Autodesk Fusion 360 part; units mm, degrees
note: some values were not read from the file. Chosen so that the rebuilt part matches the saved one: which face or edge a step refers to.
(part 3 of 3)
sketch "Sketch7" plane through (0, -7, 0) normal (0, -1, 0) x (1, 0, 0)
  circle A0 centre (0, 0) radius 34.5
  circle A1 centre (0, 0) radius 49
  line L0 (0, 34.5) -> (0, 36.5)
  line L1 (0, 36.5) -> (0, 37.03)
  line L2 (0, 37.03) -> (3.25, 37.03)
  line L3 (3.25, 37.03) -> (3.25, 34.3466)
  line L4 (-6.3382, 35.9455) -> (-6.4302, 36.4674)
  line L5 (-6.4302, 36.4674) -> (-3.2296, 37.0318)
  line L6 (-3.2296, 37.0318) -> (-2.7636, 34.3891)
  line L7 (-5.9909, 33.9759) -> (-6.3382, 35.9455)
  line L8 (-12.4837, 34.2988) -> (-12.665, 34.7968)
  line L9 (-12.665, 34.7968) -> (-9.611, 35.9084)
  line L10 (-9.611, 35.9084) -> (-8.6932, 33.3868)
  line L11 (-11.7997, 32.4194) -> (-12.4837, 34.2988)
  line L12 (-18.25, 31.6099) -> (-18.515, 32.0689)
  line L13 (-18.515, 32.0689) -> (-15.7004, 33.6939)
  line L14 (-15.7004, 33.6939) -> (-14.3587, 31.37)
  line L15 (-17.25, 29.8779) -> (-18.25, 31.6099)
  line L16 (-23.4617, 27.9606) -> (-23.8024, 28.3666)
  line L17 (-23.8024, 28.3666) -> (-21.3128, 30.4557)
  line L18 (-21.3128, 30.4557) -> (-19.5879, 28.4001)
  line L19 (-22.1762, 26.4285) -> (-23.4617, 27.9606)
  line L20 (-27.9606, 23.4617) -> (-28.3666, 23.8024)
  line L21 (-28.3666, 23.8024) -> (-26.2776, 26.2921)
  line L22 (-26.2776, 26.2921) -> (-24.2219, 24.5672)
  line L23 (-26.4285, 22.1762) -> (-27.9606, 23.4617)
  line L24 (-31.6099, 18.25) -> (-32.0689, 18.515)
  line L25 (-32.0689, 18.515) -> (-30.4439, 21.3296)
  line L26 (-30.4439, 21.3296) -> (-28.12, 19.9879)
  line L27 (-29.8779, 17.25) -> (-31.6099, 18.25)
  line L28 (-34.2988, 12.4837) -> (-34.7968, 12.665)
  line L29 (-34.7968, 12.665) -> (-33.6853, 15.719)
  line L30 (-33.6853, 15.719) -> (-31.1637, 14.8012)
  line L31 (-32.4194, 11.7997) -> (-34.2988, 12.4837)
  line L32 (-35.9455, 6.3382) -> (-36.4674, 6.4302)
  line L33 (-36.4674, 6.4302) -> (-35.9031, 9.6308)
  line L34 (-35.9031, 9.6308) -> (-33.2604, 9.1648)
  line L35 (-33.9759, 5.9909) -> (-35.9455, 6.3382)
  line L36 (-36.5, 0) -> (-37.03, 0)
  line L37 (-37.03, 0) -> (-37.03, 3.25)
  line L38 (-37.03, 3.25) -> (-34.3466, 3.25)
  line L39 (-34.5, 0) -> (-36.5, 0)
  line L40 (-35.9455, -6.3382) -> (-36.4674, -6.4302)
  line L41 (-36.4674, -6.4302) -> (-37.0318, -3.2296)
  line L42 (-37.0318, -3.2296) -> (-34.3891, -2.7636)
  line L43 (-33.9759, -5.9909) -> (-35.9455, -6.3382)
  line L44 (-34.2988, -12.4837) -> (-34.7968, -12.665)
  line L45 (-34.7968, -12.665) -> (-35.9084, -9.611)
  line L46 (-35.9084, -9.611) -> (-33.3868, -8.6932)
  line L47 (-32.4194, -11.7997) -> (-34.2988, -12.4837)
  line L48 (-31.6099, -18.25) -> (-32.0689, -18.515)
  line L49 (-32.0689, -18.515) -> (-33.6939, -15.7004)
  line L50 (-33.6939, -15.7004) -> (-31.37, -14.3587)
  line L51 (-29.8779, -17.25) -> (-31.6099, -18.25)
  line L52 (-27.9606, -23.4617) -> (-28.3666, -23.8024)
  line L53 (-28.3666, -23.8024) -> (-30.4557, -21.3128)
  line L54 (-30.4557, -21.3128) -> (-28.4001, -19.5879)
  line L55 (-26.4285, -22.1762) -> (-27.9606, -23.4617)
  line L56 (-23.4617, -27.9606) -> (-23.8024, -28.3666)
  line L57 (-23.8024, -28.3666) -> (-26.2921, -26.2776)
  line L58 (-26.2921, -26.2776) -> (-24.5672, -24.2219)
  line L59 (-22.1762, -26.4285) -> (-23.4617, -27.9606)
  line L60 (-18.25, -31.6099) -> (-18.515, -32.0689)
  line L61 (-18.515, -32.0689) -> (-21.3296, -30.4439)
  line L62 (-21.3296, -30.4439) -> (-19.9879, -28.12)
  line L63 (-17.25, -29.8779) -> (-18.25, -31.6099)
  line L64 (-12.4837, -34.2988) -> (-12.665, -34.7968)
  line L65 (-12.665, -34.7968) -> (-15.719, -33.6853)
  line L66 (-15.719, -33.6853) -> (-14.8012, -31.1637)
  line L67 (-11.7997, -32.4194) -> (-12.4837, -34.2988)
  line L68 (-6.3382, -35.9455) -> (-6.4302, -36.4674)
  line L69 (-6.4302, -36.4674) -> (-9.6308, -35.9031)
  line L70 (-9.6308, -35.9031) -> (-9.1648, -33.2604)
  line L71 (-5.9909, -33.9759) -> (-6.3382, -35.9455)
  line L72 (0, -36.5) -> (0, -37.03)
  line L73 (0, -37.03) -> (-3.25, -37.03)
  line L74 (-3.25, -37.03) -> (-3.25, -34.3466)
  line L75 (0, -34.5) -> (0, -36.5)
  line L76 (6.3382, -35.9455) -> (6.4302, -36.4674)
  line L77 (6.4302, -36.4674) -> (3.2296, -37.0318)
  line L78 (3.2296, -37.0318) -> (2.7636, -34.3891)
  line L79 (5.9909, -33.9759) -> (6.3382, -35.9455)
  line L80 (12.4837, -34.2988) -> (12.665, -34.7968)
  line L81 (12.665, -34.7968) -> (9.611, -35.9084)
  line L82 (9.611, -35.9084) -> (8.6932, -33.3868)
  line L83 (11.7997, -32.4194) -> (12.4837, -34.2988)
  line L84 (18.25, -31.6099) -> (18.515, -32.0689)
  line L85 (18.515, -32.0689) -> (15.7004, -33.6939)
  line L86 (15.7004, -33.6939) -> (14.3587, -31.37)
  line L87 (17.25, -29.8779) -> (18.25, -31.6099)
  line L88 (23.4617, -27.9606) -> (23.8024, -28.3666)
  line L89 (23.8024, -28.3666) -> (21.3128, -30.4557)
  line L90 (21.3128, -30.4557) -> (19.5879, -28.4001)
  line L91 (22.1762, -26.4285) -> (23.4617, -27.9606)
  line L92 (27.9606, -23.4617) -> (28.3666, -23.8024)
  line L93 (28.3666, -23.8024) -> (26.2776, -26.2921)
  line L94 (26.2776, -26.2921) -> (24.2219, -24.5672)
  line L95 (26.4285, -22.1762) -> (27.9606, -23.4617)
  line L96 (31.6099, -18.25) -> (32.0689, -18.515)
  line L97 (32.0689, -18.515) -> (30.4439, -21.3296)
  line L98 (30.4439, -21.3296) -> (28.12, -19.9879)
  line L99 (29.8779, -17.25) -> (31.6099, -18.25)
  line L100 (34.2988, -12.4837) -> (34.7968, -12.665)
  line L101 (34.7968, -12.665) -> (33.6853, -15.719)
  line L102 (33.6853, -15.719) -> (31.1637, -14.8012)
  line L103 (32.4194, -11.7997) -> (34.2988, -12.4837)
  line L104 (35.9455, -6.3382) -> (36.4674, -6.4302)
  line L105 (36.4674, -6.4302) -> (35.9031, -9.6308)
  line L106 (35.9031, -9.6308) -> (33.2604, -9.1648)
  line L107 (33.9759, -5.9909) -> (35.9455, -6.3382)
  line L108 (36.5, 0) -> (37.03, 0)
  line L109 (37.03, 0) -> (37.03, -3.25)
  line L110 (37.03, -3.25) -> (34.3466, -3.25)
  line L111 (34.5, 0) -> (36.5, 0)
  line L112 (35.9455, 6.3382) -> (36.4674, 6.4302)
  line L113 (36.4674, 6.4302) -> (37.0318, 3.2296)
  line L114 (37.0318, 3.2296) -> (34.3891, 2.7636)
  line L115 (33.9759, 5.9909) -> (35.9455, 6.3382)
  line L116 (34.2988, 12.4837) -> (34.7968, 12.665)
  line L117 (34.7968, 12.665) -> (35.9084, 9.611)
  line L118 (35.9084, 9.611) -> (33.3868, 8.6932)
  line L119 (32.4194, 11.7997) -> (34.2988, 12.4837)
  line L120 (31.6099, 18.25) -> (32.0689, 18.515)
  line L121 (32.0689, 18.515) -> (33.6939, 15.7004)
  line L122 (33.6939, 15.7004) -> (31.37, 14.3587)
  line L123 (29.8779, 17.25) -> (31.6099, 18.25)
  line L124 (27.9606, 23.4617) -> (28.3666, 23.8024)
  line L125 (28.3666, 23.8024) -> (30.4557, 21.3128)
  line L126 (30.4557, 21.3128) -> (28.4001, 19.5879)
  line L127 (26.4285, 22.1762) -> (27.9606, 23.4617)
  line L128 (23.4617, 27.9606) -> (23.8024, 28.3666)
  line L129 (23.8024, 28.3666) -> (26.2921, 26.2776)
  line L130 (26.2921, 26.2776) -> (24.5672, 24.2219)
  line L131 (22.1762, 26.4285) -> (23.4617, 27.9606)
  line L132 (18.25, 31.6099) -> (18.515, 32.0689)
  line L133 (18.515, 32.0689) -> (21.3296, 30.4439)
  line L134 (21.3296, 30.4439) -> (19.9879, 28.12)
  line L135 (17.25, 29.8779) -> (18.25, 31.6099)
  line L136 (12.4837, 34.2988) -> (12.665, 34.7968)
  line L137 (12.665, 34.7968) -> (15.719, 33.6853)
  line L138 (15.719, 33.6853) -> (14.8012, 31.1637)
  line L139 (11.7997, 32.4194) -> (12.4837, 34.2988)
  line L140 (6.3382, 35.9455) -> (6.4302, 36.4674)
  line L141 (6.4302, 36.4674) -> (9.6308, 35.9031)
  line L142 (9.6308, 35.9031) -> (9.1648, 33.2604)
  line L143 (5.9909, 33.9759) -> (6.3382, 35.9455)
  dimension "d60" = 3.25
  dimension "d62" = 360
  constraint coincident A0 L0.start
  constraint vertical L0
  constraint parallel L0 L1
  constraint perpendicular L1 L2
  constraint coincident A0 L3.end
  constraint perpendicular L2 L3
  measures "d60" distance of L1.end L2.end
sketch "Sketch8" plane through (-23.8024, 0, -28.3666) normal (0.642788, 0, 0.766044) x (0.766044, 0, -0.642788)
  line L0 (-3.25, -7) -> (0, -7)
  line L1 (0, -7) -> (0, 0)
  line L2 (0, 0) -> (-3.25, 0)
  line L3 (-3.25, 0) -> (-3.25, -7)
  line L4 (-3.25, -7) -> (0, -7)
  line L5 (0, -7) -> (0, -2.2084)
  line L6 (-1, -1.2084) -> (-2.25, -1.2084)
  line L7 (-3.25, -2.2084) -> (-3.25, -7)
  arc A0 (-2.25, -1.2084) -> (-3.25, -2.2084) centre (-2.25, -2.2084) ccw
  arc A1 (0, -2.2084) -> (-1, -1.2084) centre (-1, -2.2084) ccw
  dimension "d65" = 1
  dimension "d66" = 5.7916
  constraint horizontal L4
  constraint vertical L5
  constraint horizontal L6
  constraint vertical L7
  constraint tangent L6 A0
  constraint tangent L7 A0
  constraint tangent L6 A1
  constraint tangent L5 A1
  constraint equal A0 A1
  measures "d65" radius of A0
  measures "d66" distance of L4 L6
extrude "Extrude9" cut sketch "Sketch8" along normal blind 6 and the other way blind 22 contours L0 L1 L3 L4 L5 L6 L7 A0 A1
pattern_circular "C-Pattern1" count 36 over 360 about axis through (0, 1.75, 0) along (0, 1, 0) of "Extrude9"
sketch "Sketch9" plane through (0, -7, 0) normal (0, -1, 0) x (1, 0, 0)
  line L0 (0, 34.5) -> (0, 49)
  arc A0 (0, 49) -> (-5.2894, 48.7137) centre (0, 0) ccw
  line L1 (-5.2894, 48.7137) -> (-2.7636, 34.3891)
  arc A1 (0, 34.5) -> (-2.7636, 34.3891) centre (0, 0) ccw
  circle A2 centre (0, 0) radius 49.0012
  circle A3 centre (0, 0) radius 34.5
  dimension "d73" = 69
  constraint concentric A0 A2
  constraint concentric A2 A3
  measures "d73" diameter of A3
extrude "Extrude10" add sketch "Sketch9" along normal blind 1 contours L0 A0 L1 A1 A2 A3 | L0 L1 A2 A3
sketch "Sketch10" plane through (0, -8, 0) normal (0, -1, 0) x (1, 0, 0)
  circle A0 centre (0, 0) radius 34.5
  circle A1 centre (0, 0) radius 49.0012
  circle A2 centre (0, 0) radius 49.0012
  constraint concentric A0 A2
ref_plane "WorkPlane1" through (0, -15, 0) normal (0, -1, 0) x (1, 0, 0)
sketch "Sketch11" plane through (0, -15, 0) normal (0, -1, 0) x (-1, 0, 0)
  circle A0 centre (0, 0) radius 43.0116
  constraint coincident A0.centre origin
loft "Loft1" add profiles "Sketch10", "Sketch11" section 1 section 2
sketch "Sketch12" plane through (0, 0, 0) normal (0, 1, 0) x (1, 0, 0)
extrude "Extrude11" add 1 faces at (8.8126, -8, 12.9257) along direction (0, 1, 0) blind 1
